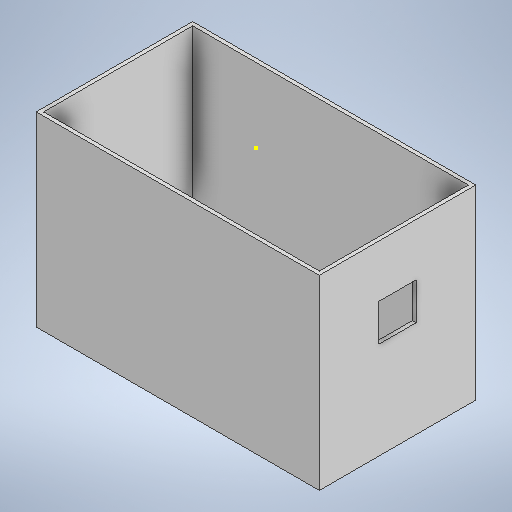
# Autodesk Inventor part: mcu_place
Saved by Autodesk Inventor 2025.2 (Build 292293000, 293)
## iProperties
Created: 2025-02-18
Part Number: mcu_place
Material: Generic
Document SubType Name: Modeling
Designer: ACER
Density: 1 g/cm^3
Appearance: Default
Author: ACER
Autodesk Inventor part; units mm, degrees
ref_plane "YZ Plane" through (0, 0, 0) normal (1, 0, 0) x (0, 1, 0)
ref_plane "XZ Plane" through (0, 0, 0) normal (0, 1, 0) x (-1, 0, 0)
ref_plane "XY Plane" through (0, 0, 0) normal (0, 0, 1) x (1, 0, 0)
sketch "Sketch1" plane through (0, 0, 0) normal (0, 1, 0) x (-1, 0, 0)
  line L0 (-38, 21) -> (38, 21)
  line L1 (38, 21) -> (38, -21)
  line L2 (38, -21) -> (-38, -21)
  line L3 (-38, -21) -> (-38, 21)
  line L4 (-38, 21) -> (38, -21) construction
  line L5 (38, 21) -> (-38, -21) construction
  point P0 (0, 0)
  dimension "d0" = 42
  dimension "d1" = 76
  constraints: 12 end point, 2 midpoint, 2 parallel, 1 horizontal, 1 perpendicular
  measures "d0" distance of L0.end L1.end
  measures "d1" distance of L1.end L2.end
extrude "Extrusion1" add sketch "Sketch1" along normal blind 50
sketch "Sketch2" plane through (0, 50, 0) normal (0, 1, 0) x (1, 0, 0)
  point P0 (0, 0)
sketch "Sketch3" plane through (0, 50, 0) normal (0, 1, 0) x (1, 0, 0)
  line L0 (-37, -20) -> (37, -20)
  line L1 (37, -20) -> (37, 20)
  line L2 (37, 20) -> (-37, 20)
  line L3 (-37, 20) -> (-37, -20)
  line L4 (-37, -20) -> (37, 20) construction
  line L5 (37, -20) -> (-37, 20) construction
  point P0 (0, 0)
  dimension "d4" = 40
  dimension "d5" = 74
  constraints: 12 end point, 2 midpoint, 2 parallel, 1 horizontal, 1 perpendicular
  measures "d4" distance of L0.end L1.end
  measures "d5" distance of L1.end L2.end
extrude "Extrusion2" cut sketch "Sketch3" against normal blind 48
sketch "Sketch4" plane through (38, 0, 21) normal (1, 0, 0) x (0, 0, -1)
  line L0 (26, 74) -> (16, 74)
  line L1 (16, 74) -> (16, 26)
  line L2 (16, 26) -> (26, 26)
  line L3 (26, 26) -> (26, 74)
  line L4 (0, 50) -> (42, 50) projected
  line L5 (26, 74) -> (16, 26) construction
  line L6 (16, 74) -> (26, 26) construction
  line L7 (16, 26) -> (26, 26)
  line L8 (26, 26) -> (26, 35.9645)
  line L9 (26, 35.9645) -> (16, 35.9645)
  line L10 (16, 35.9645) -> (16, 26)
  point P0 (21, 0)
  point P1 (21, 50)
  dimension "d8" = 10
  dimension "d9" = 48
  dimension "d10" = 10
  constraints: 20 end point, 4 parallel, 3 midpoint, 2 horizontal, 2 perpendicular, 1 point on line
  measures "d8" distance of L1.end L2.end
  measures "d9" distance of L2.end L0.start
  measures "d10" distance of L8.end L9.end
extrude "Extrusion3" cut sketch "Sketch4" against normal blind 20 contours L3 L2 L1 L9
body "Solid1"
